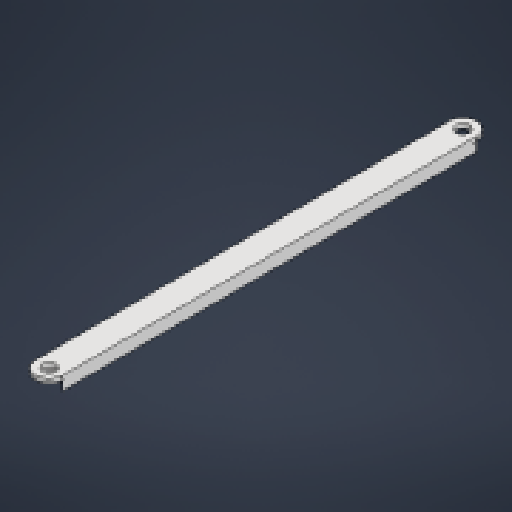
# Autodesk Inventor part: MainBar
Saved by Autodesk Inventor 2024.2 (Build 282272000, 272)
## iProperties
Created: 2023-12-28
Part Number: MainBar
Material: 一般
Document SubType Name: Modeling
Designer: Hanaoka
Density: 1 g/cm^3
Appearance: 既定
Author: Hanaoka
Autodesk Inventor part; units mm, degrees
ref_plane "YZ Plane" through (0, 0, 0) normal (1, 0, 0) x (0, 1, 0)
ref_plane "XZ Plane" through (0, 0, 0) normal (0, 1, 0) x (-1, 0, 0)
ref_plane "XY Plane" through (0, 0, 0) normal (0, 0, 1) x (1, 0, 0)
sketch "スケッチ1" plane through (0, 0, 0) normal (0, 1, 0) x (-1, 0, 0)
  line L0 (0, 49) -> (0, 49)
  line L1 (3, 46) -> (3, -46)
  line L2 (0, -49) -> (0, -49)
  line L3 (-3, -46) -> (-3, 46)
  line L4 (-3, 49) -> (3, -49) construction
  line L5 (3, 49) -> (-3, -49) construction
  arc A0 (0, -49) -> (3, -46) centre (0, -46) ccw
  arc A1 (-3, -46) -> (0, -49) centre (0, -46) ccw
  arc A2 (0, 49) -> (-3, 46) centre (0, 46) ccw
  arc A3 (3, 46) -> (0, 49) centre (0, 46) ccw
  circle A4 centre (0, 46) radius 1.5
  circle A5 centre (0, 46) radius 3 construction
  line L6 (3, 0) -> (-3, 0) construction
  circle A6 centre (0, -46) radius 1.5
  circle A7 centre (0, -46) radius 3 construction
  point P0 (0, 0)
  dimension "d0" = 3
  dimension "d1" = 98
  dimension "d2" = 6
  dimension "d3" = 3
  dimension "d4" = 6
  constraints: 14 end point, 10 tangent, 8 centre point, 8 point on circle, 8 point on line, 4 midpoint, 3 equal radius, 2 coincident, 2 parallel, 2 symmetric about line, 1 horizontal, 1 perpendicular, 2 other
  measures "d0" radius of A0
  measures "d1" distance between parallel lines of L2 L0
  measures "d2" distance between parallel lines of L3 L1
  measures "d3" diameter of A4
  measures "d4" diameter of A5
extrude "押し出し1" add sketch "スケッチ1" along normal blind 1
sketch "スケッチ2" plane through (0, 0, 0) normal (0, -1, 0) x (1, 0, 0)
  circle A0 centre (0, 46) radius 1.5 projected
  circle A1 centre (0, 46) radius 3
  circle A2 centre (0, -46) radius 1.5 projected
  circle A3 centre (0, -46) radius 3
  line L0 (3, 46) -> (3, -46) projected
  arc A4 (3, 46) -> (-3, 46) centre (0, 46) ccw projected
  line L1 (-3, -46) -> (-3, 46) projected
  arc A5 (-3, -46) -> (3, -46) centre (0, -46) ccw projected
  circle A6 centre (0, -46) radius 1.5 projected
  circle A7 centre (0, 46) radius 1.5 projected
  point P0 (0, 0)
  point P1 (-3, 46)
  point P2 (-3, -46)
  point P3 (3, -46)
  point P4 (3, 46)
  dimension "d7" = 6
  constraints: 2 centre point, 2 coincident, 1 equal radius
  measures "d7" diameter of A1
extrude "押し出し2" add sketch "スケッチ2" along normal blind 2 contours L0 A3 L1 A1
